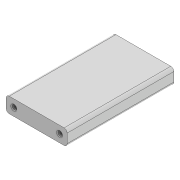
# Autodesk Inventor part: Стенка БСП
Saved by Autodesk Inventor 2022 (Build 260153000, 153)
## iProperties
Created: 2023-02-18
Part Number: Стенка БСП
Material: Типовые
Document SubType Name: Modeling
Designer: Глеб
Density: 1 g/cm^3
Appearance: По умолчанию
Mass: 26.9088 g
Surface Area: 86.7888 cm^2
Volume: 26.9088 cm^3
Author: Глеб
Autodesk Inventor part; units mm, degrees
ref_plane "YZ Plane" through (0, 0, 0) normal (1, 0, 0) x (0, 1, 0)
ref_plane "XZ Plane" through (0, 0, 0) normal (0, 1, 0) x (-1, 0, 0)
ref_plane "XY Plane" through (0, 0, 0) normal (0, 0, 1) x (1, 0, 0)
sketch "Эскиз1" plane through (0, 0, 0) normal (0, 0, 1) x (1, 0, 0)
  line L0 (18, -5) -> (-18, -5)
  line L1 (-20, -3) -> (-20, 3)
  line L2 (-18, 5) -> (18, 5)
  line L3 (20, 3) -> (20, -3)
  line L4 (20, -5) -> (-20, 5) construction
  line L5 (-20, -5) -> (20, 5) construction
  arc A0 (-18, 5) -> (-20, 3) centre (-18, 3) ccw
  arc A1 (-20, -3) -> (-18, -5) centre (-18, -3) ccw
  arc A2 (20, 3) -> (18, 5) centre (18, 3) ccw
  arc A3 (18, -5) -> (20, -3) centre (18, -3) ccw
  point P0 (0, 0)
  dimension "d0" = 40
  dimension "d1" = 10
  dimension "d2" = 2
  constraints: 12 end point, 8 point on circle, 8 point on line, 8 tangent, 4 centre point, 3 equal radius, 2 midpoint, 2 parallel, 1 horizontal, 1 perpendicular
  measures "d0" distance of L4.end L5.end
  measures "d1" distance of L5.end L4.start
  measures "d2" radius of A0
extrude "Выдавливание1" add sketch "Эскиз1" along normal mid plane 70
sketch "Эскиз2" plane through (0, 0, 35) normal (0, 0, 1) x (1, 0, 0)
  line L0 (0, 0) -> (0, 11.0353) construction
  point P0 (-15, 0)
  point P1 (15, 0)
  dimension "d5" = 30
  constraints: 2 end point, 2 horizontal alignment, 1 symmetric about line, 1 vertical
  measures "d5" distance of point (15, 0) point (-15, 0)
hole "Отверстие1" at (-15, 0, 35) at (15, 0, 35) direction (0, 0, -1) diameter 3 depth 60
chamfer "Фаска1" distance 0.5 angle 45 2 edges at (-15, 1.5, 35) (15, 1.5, 35)
